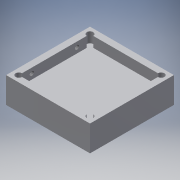
# Autodesk Inventor part: Large-cuvette-mount-50mm-V3
Saved by Autodesk Inventor 2016 (Build 200138000, 138)
## iProperties
Created: 2015-10-07
Part Number: Large-cuvette-mount-50mm-V3
Material: PC/ABS Plastic
Document SubType Name: Modeling
Designer: voigt
Density: 0.357273 g/cm^3
Appearance: Smooth - White
Author: voigt
Autodesk Inventor part; units mm, degrees
note: some values were not read from the file. Chosen so that the rebuilt part matches the saved one: direction of "Hole3".
ref_plane "YZ Plane" through (0, 0, 0) normal (1, 0, 0) x (0, 1, 0)
ref_plane "XZ Plane" through (0, 0, 0) normal (0, 1, 0) x (-1, 0, 0)
ref_plane "XY Plane" through (0, 0, 0) normal (0, 0, 1) x (1, 0, 0)
sketch "Sketch1" plane through (0, 0, 0) normal (0, 0, 1) x (1, 0, 0)
  line L0 (0, 45.5) -> (0, -45.5) construction
  line L1 (-45.5, 0) -> (45.5, 0) construction
  line L2 (-32.5, 32.5) -> (32.5, 32.5)
  line L3 (32.5, 32.5) -> (32.5, -32.5)
  line L4 (32.5, -32.5) -> (-32.5, -32.5)
  line L5 (-32.5, -32.5) -> (-32.5, 32.5)
  point P0 (0, 0)
  dimension "d0" = 65
  dimension "d1" = 65
  constraints: 8 end point, 2 parallel, 1 horizontal, 1 perpendicular, 2 other
  measures "d0" distance of L2.end L3.end
  measures "d1" distance of L3.end L4.end
extrude "Extrusion1" add sketch "Sketch1" along normal blind 20
sketch "Sketch4" plane through (0, 0, 20) normal (0, 0, 1) x (1, 0, 0)
  line L0 (-45.5, 0) -> (45.5, 0) construction
  line L1 (0, 45.5) -> (0, -45.5) construction
  line L2 (-27.55, 27.55) -> (27.55, 27.55) construction
  line L3 (27.55, 27.55) -> (27.55, -27.55) construction
  line L4 (27.55, -27.55) -> (-27.55, -27.55) construction
  line L5 (-27.55, -27.55) -> (-27.55, 27.55) construction
  point P0 (0, 0)
  dimension "d15" = 55.1
  dimension "d16" = 55.1
  constraints: 8 end point, 4 coincident, 2 parallel, 1 horizontal, 1 perpendicular, 2 other
  measures "d15" distance of L2.start L2.end
  measures "d16" distance of L4.end L2.start
hole "Hole2" at (-27.55, 27.55, 20) at (27.55, 27.55, 20) at (27.55, -27.55, 20) at (-27.55, -27.55, 20) at (-27.55, 27.55, 20) at (27.55, 27.55, 20) direction (0, 0, -1) diameter 5 depth 8
sketch "Sketch5" plane through (0, 0, 20) normal (0, 0, 1) x (1, 0, 0)
  circle A0 centre (-27.55, 27.55) radius 2.5 projected
  circle A1 centre (27.55, -27.55) radius 2.5 projected
  line L0 (-27.55, 27.55) -> (27.55, 27.55)
  line L1 (27.55, 27.55) -> (27.55, -27.55)
  line L2 (27.55, -27.55) -> (-27.55, -27.55)
  line L3 (-27.55, -27.55) -> (-27.55, 27.55)
  point P0 (0, 0)
  constraints: 8 end point, 2 parallel, 1 horizontal, 1 perpendicular
extrude "Extrusion3" cut sketch "Sketch5" against normal blind 8 contours L0 L1 A1 L2 L3 A0 | A0 L3 L0 | L1 L2 A1 picked at (-25.9042, 27.3646) picked at (27.003, -25.9868)
sketch "Sketch6" plane through (-32.5, -32.5, 0) normal (-1, 0, 0) x (0, 0, 1)
  line L0 (0, 65) -> (20, 65) projected
  line L1 (0, 0) -> (20, 0) projected
  line L2 (20, 7.45) -> (12, 7.45) construction
  line L3 (20, 57.55) -> (20, 7.45) construction
  line L4 (12, 57.55) -> (20, 57.55) construction
  line L5 (12, 7.45) -> (12, 57.55) construction
  line L6 (16, 57.55) -> (16, 7.45) construction
  point P0 (0, 32.5)
  point P1 (16, 50)
  point P2 (16, 15)
  dimension "d26" = 15
  dimension "d27" = 15
  constraints: 2 end point, 2 midpoint, 2 point on line
  measures "d26" distance from line of L1 point (16, 15)
  measures "d27" distance from line of L0 point (16, 50)
hole "Hole3" at (-32.5, 17.5, 16) at (-32.5, -17.5, 16) direction (1, 0, 0) diameter 3.242 end up to surface thread size "M4x0.7" class "6H" standard "ANSI Metric M Profile"
sketch "Sketch8" plane through (0, 0, 0) normal (0, 0, -1) x (-1, 0, 0)
  line L0 (32.5, 32.5) -> (-32.5, 32.5) construction
  line L1 (-32.5, 32.5) -> (-32.5, -32.5) construction
  line L2 (-32.5, -32.5) -> (32.5, -32.5) construction
  line L3 (32.5, -32.5) -> (32.5, 32.5) construction
  line L4 (0, -45.5) -> (0, 45.5) construction
  line L5 (-45.5, 0) -> (45.5, 0) construction
  line L6 (12.5, -12.5) -> (-12.5, -12.5)
  line L7 (-12.5, -12.5) -> (-12.5, 12.5)
  line L8 (-12.5, 12.5) -> (12.5, 12.5)
  line L9 (12.5, 12.5) -> (12.5, -12.5)
  point P0 (0, 0)
  dimension "d44" = 25
  dimension "d45" = 25
  constraints: 8 end point, 2 parallel, 1 horizontal, 1 perpendicular, 2 other
  measures "d44" distance of L6.start L6.end
  measures "d45" distance of L6.end L7.end
extrude "Extrusion4" cut sketch "Sketch8" against normal blind 6
sketch "Sketch9" plane through (0, 0, 0) normal (0, 0, -1) x (-1, 0, 0)
  line L0 (12.5, 12.5) -> (12.5, -12.5) construction
  line L1 (12.5, -12.5) -> (-12.5, -12.5) construction
  line L2 (-12.5, -12.5) -> (-12.5, 12.5) construction
  line L3 (-12.5, 12.5) -> (12.5, 12.5) construction
  line L4 (32.5, 32.5) -> (-32.5, 32.5) construction
  line L5 (-32.5, 32.5) -> (-32.5, -32.5) construction
  line L6 (-32.5, -32.5) -> (32.5, -32.5) construction
  line L7 (32.5, -32.5) -> (32.5, 32.5) construction
  line L8 (12.5, -12.5) -> (-12.5, -12.5) construction
  point P0 (0, 0)
  constraints: 4 coincident
hole "Hole5" at (-12.5, -12.5, 0) at (12.5, -12.5, 0) at (12.5, 12.5, 0) at (-12.5, 12.5, 0) direction (0, 0, 1) diameter 3 depth 6
sketch "Sketch10" plane through (0, 0, 6) normal (0, 0, -1) x (-1, 0, 0)
  point P0 (0, 0)
  point P1 (0, 0)
  constraints: 1 coincident
hole "Hole6" at (0, 0, 6) direction (0, 0, 1) diameter 3.242 depth 4 tip angle 118 thread size "M4x0.7" class "6H" standard "ANSI Metric M Profile"
body "Solid1"
